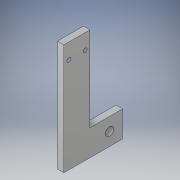
# Autodesk Inventor part: PaddleCollection2.1ServoSupport
Saved by Autodesk Inventor 2019 (Build 230136000, 136)
## iProperties
Created: 2018-10-23
Part Number: PaddleCollection2.1ServoSupport
Material: Aluminum 6061
Document SubType Name: Modeling
Designer: User
Density: 2.7 g/cm^3
Appearance: Aluminum - Flat
Author: User
Autodesk Inventor part; units mm, degrees
ref_plane "YZ Plane" through (0, 0, 0) normal (1, 0, 0) x (0, 1, 0)
ref_plane "XZ Plane" through (0, 0, 0) normal (0, 1, 0) x (-1, 0, 0)
ref_plane "XY Plane" through (0, 0, 0) normal (0, 0, 1) x (1, 0, 0)
sketch "Sketch1" plane through (0, 0, 0) normal (1, 0, 0) x (0, 1, 0)
  line L0 (0, 0) -> (107.95, 0)
  line L1 (107.95, 0) -> (107.95, -57.15)
  line L2 (107.95, -57.15) -> (0, -57.15)
  line L3 (0, -57.15) -> (0, 0)
  line L4 (107.95, -57.15) -> (25.4, -57.15)
  line L5 (25.4, -57.15) -> (25.4, -25.4)
  line L6 (25.4, -25.4) -> (107.95, -25.4)
  line L7 (107.95, -25.4) -> (107.95, -57.15)
  dimension "d0" = 107.95
  dimension "d1" = 57.15
  dimension "d2" = 82.55
  dimension "d3" = 31.75
  constraints: 16 end point, 4 parallel, 2 horizontal, 2 perpendicular
  measures "d0" distance of L1.end L2.end
  measures "d1" distance of L0.end L1.end
  measures "d2" distance of L5.end L6.end
  measures "d3" distance of L4.end L5.end
extrude "Extrusion1" add sketch "Sketch1" along normal blind 6.35 contours L0 L1 L6 L5 L2 L3
sketch "Sketch2" plane through (6.35, 0, 0) normal (1, 0, 0) x (0, 0, -1)
  line L0 (0, 0) -> (57.15, 0) projected
  line L1 (57.15, 25.4) -> (25.4, 25.4) projected
  line L2 (25.4, 25.4) -> (25.4, 107.95) projected
  line L3 (25.4, 107.95) -> (0, 107.95) projected
  line L4 (0, 107.95) -> (0, 0) projected
  line L5 (0, 0) -> (57.15, 0) projected
  line L6 (57.15, 0) -> (57.15, 25.4) projected
  point P0 (4.699, 92.9894)
  point P1 (20.701, 92.9894)
  dimension "d6" = 92.9894
  dimension "d7" = 92.9894
  dimension "d8" = 16.002
  dimension "d9" = 25.4
  dimension "d10" = 4.699
  measures "d6" distance from line of L0 point (4.699, 92.989)
  measures "d7" distance from line of L0 point (20.701, 92.989)
  measures "d8" distance of point (20.701, 92.989) point (4.699, 92.989)
  measures "d9" distance of L2.end L3.end
  measures "d10" distance from line of L4 point (4.699, 92.989)
hole "Hole1" at (6.35, 92.9894, -4.699) at (6.35, 92.9894, -20.701) direction (-1, 0, 0) diameter 3.81 end through all
sketch "Sketch3" plane through (6.35, 0, 0) normal (1, 0, 0) x (0, 0, -1)
  line L0 (57.15, 25.4) -> (25.4, 25.4) projected
  line L1 (57.15, 0) -> (57.15, 25.4) projected
  point P0 (0, 0)
  point P1 (44.45, 12.7)
  dimension "d18" = 12.7
  dimension "d19" = 12.7
  measures "d18" distance from line of L0 point (44.45, 12.7)
  measures "d19" distance from line of L1 point (44.45, 12.7)
hole "Hole2" at (6.35, 12.7, -44.45) direction (-1, 0, 0) diameter 8.128 end through all
equation "\"d7\" = d6"
equation "\"d10\" = -0.5 * d8 + 0.5 * d9"
body "Solid1"
